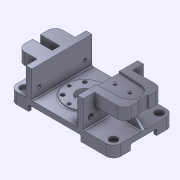
# Autodesk Inventor part: 18102021-002-10
Saved by Autodesk Inventor 2021 (Build 250183000, 183)
## iProperties
Created: 2021-10-17
Part Number: 18102021-002-10
Material: Iron, Cast
Document SubType Name: Modeling
Designer: DuctopwH
Density: 7.15 g/cm^3
Appearance: Iron Gray
Author: DuctopwH
Autodesk Inventor part; units mm, degrees
ref_plane "YZ Plane" through (0, 0, 0) normal (1, 0, 0) x (0, 1, 0)
ref_plane "XZ Plane" through (0, 0, 0) normal (0, 1, 0) x (-1, 0, 0)
ref_plane "XY Plane" through (0, 0, 0) normal (0, 0, 1) x (1, 0, 0)
sketch "Sketch1" plane through (0, 0, 0) normal (0, 1, 0) x (-1, 0, 0)
  line L0 (-79.5, 46) -> (79.5, 46)
  line L1 (79.5, 46) -> (79.5, -46)
  line L2 (79.5, -46) -> (-79.5, -46)
  line L3 (-79.5, -46) -> (-79.5, 46)
  line L4 (-79.5, 46) -> (79.5, -46) construction
  line L5 (79.5, 46) -> (-79.5, -46) construction
  point P0 (0, 0)
  dimension "d0" = 92
  dimension "d1" = 159
  constraints: 12 end point, 2 midpoint, 2 parallel, 1 horizontal, 1 perpendicular
  measures "d0" distance between parallel lines of L0 L2
  measures "d1" distance of L1.end L2.end
extrude "Extrusion1" add sketch "Sketch1" along normal blind 17
sketch "Sketch2" plane through (-79.5, 0, 46) normal (0, 0, 1) x (1, 0, 0)
  line L0 (25, 0) -> (34, 0)
  line L1 (34, 0) -> (34, 59)
  line L2 (34, 59) -> (25, 59)
  line L3 (25, 59) -> (25, 0)
  line L4 (159, 0) -> (0, 0) projected
  line L5 (104, 0) -> (113, 0)
  line L6 (113, 0) -> (113, 59)
  line L7 (113, 59) -> (104, 59)
  line L8 (104, 59) -> (104, 0)
  line L9 (159, 0) -> (159, 17) projected
  line L10 (0, 0) -> (0, 17) projected
  point P0 (79.5, 0)
  point P1 (79.5, 0)
  dimension "d4" = 55
  dimension "d5" = 46
  dimension "d6" = 9
  dimension "d7" = 25
  dimension "d8" = 59
  constraints: 16 end point, 4 parallel, 3 point on line, 2 horizontal, 2 perpendicular, 1 midpoint
  measures "d4" distance between parallel lines of L9 L8
  measures "d5" distance between parallel lines of L9 L6
  measures "d6" distance between parallel lines of L3 L1
  measures "d7" distance between parallel lines of L10 L3
  measures "d8" distance between parallel lines of L4 L2
extrude "Extrusion2" add sketch "Sketch2" against normal up to surface (92 mm away)
sketch "Sketch3" plane through (-54.5, 59, 46) normal (0, 1, 0) x (1, 0, 0)
  line L0 (54.5, 46) -> (0, 46)
  line L1 (0, 0) -> (0, 92) projected
  line L2 (0, 75) -> (-19, 75)
  line L3 (-30, 64) -> (-30, 52)
  line L4 (-30, 52) -> (0, 52)
  line L5 (0, 17) -> (-19, 17)
  line L6 (-30, 28) -> (-30, 40)
  line L7 (-30, 40) -> (0, 40)
  arc A0 (-19, 75) -> (-30, 64) centre (-19, 64) ccw
  arc A1 (-30, 28) -> (-19, 17) centre (-19, 28) ccw
  circle A2 centre (-11.54, 11) radius 6
  circle A3 centre (-11.54, 81) radius 6
  point P0 (-30, 75)
  point P1 (-30, 17)
  point P2 (0, 17)
  point P3 (0, 40)
  dimension "d11" = 30
  dimension "d12" = 12
  dimension "d13" = 11
  dimension "d16" = 70
  dimension "d17" = 12
  constraints: 14 end point, 6 point on line, 5 symmetric about line, 5 tangent, 4 centre point, 4 point on circle, 2 perpendicular, 1 equal radius, 1 horizontal, 1 midpoint, 1 other
  measures "d11" distance of L3.end L4.end
  measures "d12" distance between parallel lines of L7 L4
  measures "d13" radius of A0
  measures "d16" distance of A2.centre A3.centre
  measures "d17" diameter of A2
extrude "Extrusion3" add sketch "Sketch3" against normal blind 18 contours L5 A1 L6 L7 L1 | L4 L3 A0 L2 L1
sketch "Sketch4" plane through (-84.5, 59, -6) normal (0, 0, 1) x (1, 0, 0)
  line L0 (30, -42) -> (5, -42) projected
  line L1 (0, -18) -> (5, -42)
  line L2 (30, -18) -> (0, -18) projected
  line L3 (30, 0) -> (30, -42) projected
  circle A0 centre (12, -29) radius 3
  line L4 (39, -42) -> (39, 0) projected
  line L5 (0, 0) -> (30, 0) projected
  line L6 (0, 0) -> (0, -18) projected
  point P0 (84.5, -59)
  dimension "d18" = 6
  dimension "d19" = 27
  dimension "d20" = 29
  constraints: 2 end point, 1 centre point
  measures "d18" diameter of A0
  measures "d19" distance from line of L4 A0.centre
  measures "d20" distance from line of L5 A0.centre
extrude "Extrusion4" add sketch "Sketch4" against normal blind 4 contours L0 L1 L2 L3
mirror "Mirror1" about plane through (0, 0, 0) normal (0, 0, 1) of "Extrusion4"
fillet "Fillet1" radius 2 10 edges at (-54.5, 41, -19.5) (-69.5, 41, -10) (-54.5, 29, -10) (-54.5, 17, -28) (-67, 17, -10) (-54.5, 17, 28) (-67, 17, 10) (-54.5, 29, 10) (-69.5, 41, 10) (-54.5, 41, 19.5)
sketch "Sketch7" plane through (-54.5, 59, 29) normal (-1, 0, 0) x (0, 0, 1)
  circle A0 centre (6, -29) radius 6
  line L0 (-23, 0) -> (-35, 0) projected
  line L1 (-29, 0) -> (-29, -59)
  circle A1 centre (-64, -29) radius 6
  line L2 (17, 0) -> (0, 0) projected
  line L3 (0, 0) -> (0, -18) projected
  circle A2 centre (-64, -29) radius 2.5
  circle A3 centre (6, -29) radius 2.5
  dimension "d27" = 70
  dimension "d28" = 29
  dimension "d30" = 5
  constraints: 4 centre point, 2 end point, 2 symmetric about line, 1 coincident, 1 midpoint, 1 tangent, 1 vertical, 2 other
  measures "d27" distance of A1.centre A0.centre
  measures "d28" distance from line of A0.centre L2
  measures "d30" diameter of A3
extrude "Extrusion6" cut sketch "Sketch7" against normal through all contours A2 | A3
sketch "Sketch8" plane through (-54.5, 59, 29) normal (-1, 0, 0) x (0, 0, 1)
  circle A0 centre (-64, -29) radius 2.5 projected
  circle A1 centre (-64, -29) radius 4
  circle A2 centre (6, -29) radius 2.5 projected
  circle A3 centre (6, -29) radius 4
  point P0 (-29, -59)
  dimension "d33" = 8
  constraints: 2 centre point, 2 coincident, 1 equal radius
  measures "d33" diameter of A1
extrude "Extrusion7" cut sketch "Sketch8" against normal blind 3 contours A0 | A1 | A2 | A3
sketch "Sketch9" plane through (33.5, 17, 46) normal (1, 0, 0) x (0, 0, -1)
  circle A0 centre (11, 13) radius 2.5 projected
  circle A1 centre (11, 13) radius 4
  circle A2 centre (81, 13) radius 2.5 projected
  circle A3 centre (81, 13) radius 4
  circle A4 centre (11, 13) radius 4 projected
  point P0 (46, -17)
  constraints: 2 centre point, 2 coincident, 2 equal radius
extrude "Extrusion8" cut sketch "Sketch9" against normal blind 3 contours A0 | A1 | A2 | A3
sketch "Sketch10" plane through (-84.5, 59, -6) normal (0, 0, 1) x (1, 0, 0)
  line L0 (0, 0) -> (0, -18) projected
  circle A0 centre (0, -9) radius 30
  line L1 (30, 0) -> (30, -42) projected
  line L2 (0, -18) -> (5, -42) projected
  line L3 (4.3102, -38.6888) -> (5, -42)
  line L4 (30, -42) -> (5, -42) projected
  point P0 (84.5, -59)
  point P1 (30, -9)
  point P2 (4.3102, -38.6888)
  dimension "d38" = 60
  constraints: 2 end point, 1 collinear, 1 midpoint, 3 other
extrude "Extrusion9" add sketch "Sketch10" along normal up to surface (12 mm away) contours L1 L4 L2 A0
sketch "Sketch11" plane through (0, 17, 0) normal (0, 1, 0) x (1, 0, 0)
  line L0 (0, 0) -> (73.1994, 0)
  circle A0 centre (-68.5, -35) radius 6
  circle A1 centre (-68.5, -35) radius 2.8657
  circle A2 centre (-68.5, 35) radius 6
  circle A3 centre (-68.5, 35) radius 2.8657
  line L1 (0, 0) -> (0, -46.4979)
  circle A4 centre (68.5, -35) radius 6
  circle A5 centre (68.5, -35) radius 2.8657
  circle A6 centre (68.5, 35) radius 2.8657
  circle A7 centre (68.5, 35) radius 6
  dimension "d41" = 70
  dimension "d42" = 137
  dimension "d43" = 12
  constraints: 8 centre point, 6 symmetric about line, 4 coincident, 4 end point, 1 horizontal, 1 vertical, 6 other
  measures "d41" distance of A0.centre A3.centre
  measures "d42" distance of A0.centre A4.centre
  measures "d43" diameter of A0
extrude "Extrusion10" cut sketch "Sketch11" against normal blind 6 contours A0 | A1 | A2 | A3 | A4 | A5 | A6 | A7
sketch "Sketch12" plane through (-68.5, 11, 35) normal (0, 1, 0) x (1, 0, 0)
  circle A0 centre (0, 0) radius 6 projected
  circle A1 centre (0, 0) radius 3
  line L0 (-11.0165, 35) -> (148, 35)
  line L1 (148, -11) -> (148, 81) projected
  line L2 (68.5, 35) -> (68.5, -11)
  circle A2 centre (0, 70) radius 3
  circle A3 centre (137, 0) radius 3
  circle A4 centre (137, 70) radius 3
  dimension "d111" = 6
  constraints: 4 centre point, 4 end point, 3 symmetric about line, 1 coincident, 1 horizontal, 1 midpoint, 1 vertical, 3 other
  measures "d111" diameter of A2
extrude "Extrusion11" cut sketch "Sketch12" against normal through all contours A1 | A2 | A3 | A4
sketch "Sketch14" plane through (0, 0, 0) normal (0, -1, 0) x (1, 0, 0)
  point P0 (0, 0)
fillet "Fillet2" radius 11 4 edges at (-79.5, 8.5, 46) (79.5, 8.5, 46) (-79.5, 8.5, -46) (79.5, 8.5, -46)
sketch "Sketch15" plane through (0, 0, 0) normal (0, -1, 0) x (1, 0, 0)
  arc A0 (68.5, -46) -> (79.5, -35) centre (68.5, -35) ccw projected
  line L0 (79.5, 35) -> (79.5, -35) projected
  arc A1 (79.5, 35) -> (68.5, 46) centre (68.5, 35) ccw projected
  line L1 (-68.5, 46) -> (68.5, 46) projected
  arc A2 (-68.5, 46) -> (-79.5, 35) centre (-68.5, 35) ccw projected
  line L2 (-79.5, -35) -> (-79.5, 35) projected
  arc A3 (-79.5, -35) -> (-68.5, -46) centre (-68.5, -35) ccw projected
  line L3 (68.5, -46) -> (-68.5, -46) projected
  circle A4 centre (68.5, -35) radius 3 projected
  circle A5 centre (68.5, 35) radius 3 projected
  circle A6 centre (-68.5, -35) radius 3 projected
  circle A7 centre (-68.5, 35) radius 3 projected
  arc A8 (-68.5, 42) -> (-75.5, 35) centre (-68.5, 35) ccw
  line L4 (-68.5, 42) -> (68.5, 42)
  arc A9 (75.5, 35) -> (68.5, 42) centre (68.5, 35) ccw
  line L5 (75.5, 35) -> (75.5, -35)
  arc A10 (68.5, -42) -> (75.5, -35) centre (68.5, -35) ccw
  line L6 (68.5, -42) -> (-68.5, -42)
  arc A11 (-75.5, -35) -> (-68.5, -42) centre (-68.5, -35) ccw
  line L7 (-75.5, -35) -> (-75.5, 35)
  line L8 (-50.5, 46) -> (-50.5, -46)
  line L9 (68.5, -46) -> (-68.5, -46) projected
  line L10 (-79.5, 12) -> (-79.5, 35) projected
  line L11 (-79.5, 20) -> (79.5, 20)
  line L12 (79.5, 35) -> (79.5, -35) projected
  line L13 (0, 0) -> (79.5, 0)
  line L14 (-79.5, -20) -> (79.5, -20)
  line L15 (-68.5, 46) -> (68.5, 46) projected
  line L16 (29.5, 46) -> (29.5, -46)
  point P0 (75.5, 20)
  point P1 (29.5, 42)
  point P2 (-50.5, 42)
  point P3 (-75.5, 20)
  point P4 (-75.5, -20)
  point P5 (-50.5, -42)
  point P6 (-50.5, -46)
  point P7 (29.5, -42)
  point P8 (75.5, -20)
  dimension "d52" = 4
  dimension "d53" = 29
  dimension "d54" = 26
  dimension "d55" = 50
  constraints: 18 end point, 8 point on circle, 6 point on line, 4 centre point, 3 perpendicular, 2 symmetric about line, 1 midpoint, 7 other
  measures "d52" distance between parallel lines of L2 L7
  measures "d53" distance between parallel lines of L2 L8
  measures "d54" distance between parallel lines of L1 L11
  measures "d55" distance between parallel lines of L12 L16
extrude "Extrusion12" cut sketch "Sketch15" against normal blind 9 contours L3 L8 L6 L16 | L14 L5 L13 L0 | L16 L14 L5 A10 L6 | L6 L8 L14 L16 | L13 L5 L11 L0 | L14 L16 L13 L5 | L6 A11 L7 L14 L8 | L14 L8 L11 L16 | L13 L16 L11 L5 | L14 L7 L11 L8 | L11 L16 L4 A9 L5 | L2 L11 L7 L14 | L11 L7 A8 L4 L8 | L8 L4 L16 L11 | L8 L1 L16 L4
sketch "Sketch16" plane through (0, 17, 0) normal (0, 1, 0) x (1, 0, 0)
  line L0 (-45.5, 46) -> (-45.5, -46) projected
  line L1 (-45.5, 0) -> (24.5, 0)
  circle A0 centre (-10.5, 0) radius 29
  line L2 (24.5, -46) -> (24.5, 46) projected
  point P0 (0, 0)
  dimension "d58" = 58
  constraints: 3 midpoint, 2 end point, 1 centre point, 1 coincident, 1 horizontal
  measures "d58" diameter of A0
extrude "Extrusion13" add sketch "Sketch16" along normal blind 2
fillet "Fillet3" radius 2 1 edges at (-39.5, 17, 0)
sketch "Sketch17" plane through (-10.5, 19, 0) normal (0, 1, 0) x (1, 0, 0)
  circle A0 centre (0, 0) radius 29 projected
  circle A1 centre (0, 0) radius 24
  circle A2 centre (-24, 0) radius 2.5
  line L0 (0, 0) -> (-16.9706, 16.9706)
  line L1 (0, 0) -> (-26.5, 0)
  circle A3 centre (-16.9706, 16.9706) radius 3
  circle A4 centre (-16.9706, -16.9706) radius 3
  circle A5 centre (0, -24) radius 2.5
  circle A6 centre (16.9706, -16.9706) radius 3
  circle A7 centre (24, 0) radius 2.5
  circle A8 centre (16.9706, 16.9706) radius 3
  circle A9 centre (0, 24) radius 2.5
  circle A10 centre (0, 0) radius 12.5
  point P0 (10.5, 0)
  point P1 (0, -26.5)
  point P2 (26.5, 0)
  point P3 (0, 26.5)
  dimension "d66" = 5
  dimension "d62" = 48
  dimension "d63" = 45
  dimension "d65" = 6
  dimension "d69" = 360
  dimension "d71" = 25
  constraints: 6 centre point, 4 end point, 3 coincident, 2 horizontal alignment, 2 point on circle, 2 vertical alignment, 1 horizontal, 1 point on line, 29 other
  measures "d62" diameter of A1
  measures "d63" angle of L1 L0
  measures "d65" diameter of A3
  measures "d71" diameter of A10
extrude "Extrusion14" cut sketch "Sketch17" against normal through all contours A1 A7 | A1 A7 | A8 A1 | A1 A8 | A6 A1 | A1 A6 | A9 A1 | A1 A9 | A5 A1 | A1 A5 | A3 L0 A1 | A1 A3 | A4 A1 | A1 A4 | L0 A3 A1 | A2 L1 A1 | A1 L1 A2 | A2 L1 A1 | A1 L1 A2 | A10 L1 L0 | L0 L1 A10
sketch "Sketch18" plane through (0, 9, 0) normal (0, -1, 0) x (1, 0, 0)
  circle A0 centre (-10.5, 24) radius 2.5 projected
  circle A1 centre (-10.5, 24) radius 7
  circle A2 centre (-10.5, 0) radius 12.5 projected
  circle A3 centre (-34.5, 0) radius 7
  circle A4 centre (-10.5, -24) radius 7
  circle A5 centre (13.5, 0) radius 7
  circle A6 centre (-34.5, 0) radius 2.5 projected
  circle A7 centre (13.5, 0) radius 2.5 projected
  circle A8 centre (-10.5, -24) radius 2.5 projected
  point P0 (0, 0)
  dimension "d76" = 360
  dimension "d78" = 14
  constraints: 4 centre point, 1 coincident, 9 other
  measures "d78" diameter of A3
extrude "Extrusion15" add sketch "Sketch18" along normal blind 3 contours A1 | A3 | A4 | A5
fillet "Fillet4" radius 2 4 edges at (-17.5, 9, 24) (6.5, 9, 0) (-41.5, 9, 0) (-17.5, 9, -24)
sketch "Sketch19" plane through (24.5, 59, 46) normal (0, 1, 0) x (1, 0, 0)
  line L0 (9, 0) -> (9, 92) projected
  line L1 (9, 46) -> (53, 46)
  line L2 (53, 46) -> (53, 53.5)
  line L3 (53, 53.5) -> (55, 53.5)
  line L4 (55, 28) -> (55, 64)
  line L5 (55, 11) -> (55, 81) projected
  line L6 (44, 75) -> (9, 75)
  line L7 (53, 46) -> (53, 38.5)
  line L8 (55, 38.5) -> (55, 17)
  line L9 (44, 17) -> (9, 17)
  line L10 (53, 38.5) -> (55, 38.5)
  line L11 (-79, 75) -> (-98, 75) projected
  arc A0 (44, 17) -> (55, 28) centre (44, 28) ccw
  arc A1 (55, 64) -> (44, 75) centre (44, 64) ccw
  point P0 (-24.5, 46)
  point P1 (55, 75)
  point P2 (55, 38.5)
  dimension "d84" = 11
  dimension "d90" = 15
  dimension "d91" = 2
  constraints: 18 end point, 5 point on line, 4 point on circle, 4 symmetric about line, 4 tangent, 3 collinear, 3 perpendicular, 2 centre point, 1 equal radius, 1 horizontal, 1 midpoint
  measures "d84" radius of A0
  measures "d90" distance between parallel lines of L10 L3
  measures "d91" distance between parallel lines of L4 L2
extrude "Extrusion16" add sketch "Sketch19" against normal blind 18 contours L0 L1 L7 L10 L4 A0 L9 | L0 L6 A1 L4 L3 L2 L1
sketch "Sketch20" plane through (0, 0, 0) normal (0, 0, 1) x (1, 0, 0)
  line L0 (68.5, 17) -> (79.5, 17) projected
  line L1 (79.5, 17) -> (56.5, 41)
  line L2 (68.5, 41) -> (33.5, 41) projected
  line L3 (79.5, 59) -> (79.5, 41) projected
  line L4 (33.5, 17) -> (33.5, 59) projected
  line L5 (33.5, 17) -> (68.5, 17) projected
  line L6 (68.5, 17) -> (79.5, 17) projected
  point P0 (0, 0)
  dimension "d85" = 23
  constraints: 2 end point, 1 coincident, 1 point on line
  measures "d85" distance from line of L3 point (56.5, 41)
extrude "Extrusion17" add sketch "Sketch20" along normal mid plane 4
fillet "Fillet5" radius 2 10 edges at (56.5, 17, 2) (33.5, 17, 24) (33.5, 29, 2) (33.5, 29, -2) (33.5, 17, -24) (56.5, 17, -2) (33.5, 41, -15.5) (45, 41, -2) (33.5, 41, 15.5) (45, 41, 2)
fillet "Fillet6" radius 2 2 edges at (-45.5, 17, 0) (24.5, 17, 0)
sketch "Sketch21" plane through (24.5, 59, 46) normal (0, 1, 0) x (1, 0, 0)
  line L0 (0, 0) -> (0, 92) projected
  line L1 (0, 46) -> (60.0298, 46)
  line L2 (0, 63.7475) -> (34.8116, 61.9794)
  circle A0 centre (34, 46) radius 16
  line L3 (0, 28.2525) -> (34.8116, 30.0206)
  circle A1 centre (-18.0294, 62.9706) radius 3 projected
  circle A2 centre (-18.0294, 29.0294) radius 3 projected
  circle A3 centre (-35, 46) radius 12.5 projected
  line L4 (-35, 46) -> (-35, 65.5)
  circle A4 centre (-35, 46) radius 19.5
  line L5 (0, 63.7475) -> (-34.0109, 65.4749)
  line L6 (0, 28.2525) -> (-34.0109, 26.5251)
  point P0 (-24.5, 46)
  point P1 (34.8116, 30.0206)
  dimension "d92" = 32
  dimension "d94" = 69
  dimension "d106" = 39
  constraints: 12 end point, 3 symmetric about line, 2 point on circle, 2 point on line, 1 centre point, 1 coincident, 1 collinear, 1 horizontal, 1 midpoint, 1 tangent, 1 vertical, 4 other
  measures "d94" distance of point (34, 46) L4.start
  measures "d106" diameter of A4
extrude "Extrusion18" cut sketch "Sketch21" against normal blind 2.5 contours L0 L1 A0 L3 | L0 L2 A0 L1 | A0 L1 | A0 L1
sketch "Sketch22" plane through (24.5, 56.5, 46) normal (0, 1, 0) x (1, 0, 0)
  arc A0 (34.8116, 30.0206) -> (34.8116, 61.9794) centre (34, 46) ccw projected
  circle A1 centre (34, 46) radius 6.7051
  line L0 (34, 46) -> (11.5, 46)
  circle A2 centre (11.5, 46) radius 4.342
  point P0 (-24.5, 46)
  dimension "d98" = 22.5
  constraints: 2 centre point, 2 coincident, 2 end point, 1 horizontal
  measures "d98" distance of L0.start L0.end
hole "Hole1" at (36, 56.5, 0) at (58.5, 56.5, 0) direction (0, -1, 0) diameter 3.4587 depth 12 tip angle 118 thread size "M4x0.5" class "6H" standard "ANSI Metric M Profile"
fillet "Fillet7" radius 2 20 edges at (-59.5, 9, 42) (-75.5, 9, 27.5) (-73.4497, 9, 39.9497) (-73.4497, 9, -39.9497) (-59.5, 9, -42) (-75.5, 9, -27.5) (73.4497, 9, 39.9497) (75.5, 9, 27.5) (49, 9, 42) (73.4497, 9, -39.9497) (49, 9, -42) (75.5, 9, -27.5) (-77.5, 9, 20) (77.5, 9, 20) (-50.5, 9, 44) (-50.5, 9, -44) (77.5, 9, -20) (-77.5, 9, -20) (29.5, 9, 44) (29.5, 9, -44)
chamfer "Chamfer1" distance 1 angle 45 2 edges at (36, 56.5, -1.7294) (58.5, 56.5, -1.7294)
sketch "Sketch23" plane through (24.5, 59, 46) normal (0, 1, 0) x (1, 0, 0)
  line L0 (-129.9635, 46) -> (74.9123, 46)
  line L1 (74.9123, 46) -> (74.9123, -18.51)
  line L2 (74.9123, -18.51) -> (-129.9635, -18.51)
  line L3 (-129.9635, -18.51) -> (-129.9635, 46)
  point P0 (-24.5, 46)
  constraints: 8 end point, 2 parallel, 1 horizontal, 1 perpendicular
body "Solid1"
